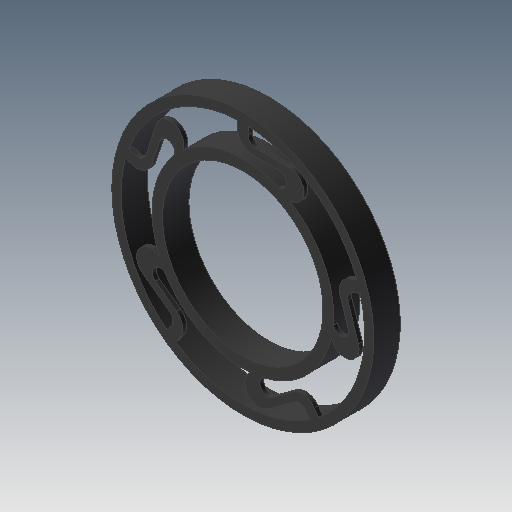
# Autodesk Inventor part: 01_Autofocus_CCTV12mm_spring_1
Saved by Autodesk Inventor 2019.4 (Build 234330000, 330)
## iProperties
Created: 2020-10-23
Part Number: 01_Autofocus_CCTV12mm_spring_1
Material: Generic
Document SubType Name: Modeling
Designer: diederichbenedict
Density: 1 g/cm^3
Appearance: Default
Author: diederichbenedict
Autodesk Inventor part; units mm, degrees
ref_plane "YZ Plane" through (0, 0, 0) normal (1, 0, 0) x (0, 1, 0)
ref_plane "XZ Plane" through (0, 0, 0) normal (0, 1, 0) x (-1, 0, 0)
ref_plane "XY Plane" through (0, 0, 0) normal (0, 0, 1) x (1, 0, 0)
ref_plane "Work Plane1" through (-22.2084, -34.255, 31.6599) normal (0, 0, 1) x (-1, 0, 0)
sketch "Sketch1" plane through (-22.2084, -34.255, 31.6599) normal (0, 0, 1) x (-1, 0, 0)
  circle A0 centre (0, 0) radius 10.2 construction
  circle A1 centre (0, 0) radius 9.25 projected
  circle A2 centre (0, 0) radius 6 projected
  circle A3 centre (0, 0) radius 6.1
  circle A4 centre (0, 0) radius 6.9
  circle A5 centre (0, 0) radius 9.95
  point P0 (-22.2084, -34.255)
  dimension "d0" = 12.2
  dimension "d1" = 0.8
  dimension "d10" = 19.9
  constraints: 3 centre point, 2 coincident
  measures "d0" diameter of A3
  measures "d1" radial gap between concentric circles of A3 A4
  measures "d10" diameter of A5
extrude "Extrusion1" add sketch "Sketch1" along normal blind 2 contours A4 | A5
sketch "Sketch2" plane through (-22.2084, -34.255, 33.6599) normal (0, 0, 1) x (1, 0, 0)
  circle A0 centre (0, 0) radius 6.1 construction
  circle A1 centre (0, 0) radius 6.9 construction
  circle A2 centre (0, 0) radius 9.25 construction
  circle A3 centre (0, 0) radius 9.25 construction
  line L0 (0.1042, 9.2494) -> (0.1042, 8.4994) construction
  circle A4 centre (0, 0) radius 6.9 construction
  line L1 (2.7219, 7.5216) -> (0.0969, 7.5216) construction
  line L2 (0.0969, 7.5216) -> (0.0969, 6.8993) construction
  line L3 (2.7219, 7.5216) -> (0.7649, 7.5216)
  line L4 (0.4969, 6.9) -> (0.4969, 6.8821)
  line L5 (3.5597, 8.0734) -> (0.9724, 8.0734)
  line L6 (0.4, 8.6458) -> (0.4, 9.2413)
  arc A5 (0.4969, 6.8821) -> (0.4969, 6.8821) centre (1.2774, -5.4017) ccw
  line L7 (-16.3817, 34.255) -> (28.6401, 34.255) projected
  arc A6 (3.5597, 5.9109) -> (3.5597, 8.0734) centre (3.5597, 6.9921) ccw
  arc A7 (2.7219, 6.3404) -> (2.7219, 7.5216) centre (2.7219, 6.931) ccw
  line L8 (-0.4, 9.0413) -> (-0.4, 9.2413)
  arc A8 (3.5597, 5.9109) -> (2.7219, 6.3404) centre (0, 0) ccw
  arc A9 (0.4, 9.2413) -> (-0.4, 9.2413) centre (0, 0) ccw
  arc A10 (3.5597, 5.9109) -> (2.3926, 6.4719) centre (0, 0) ccw construction
  arc A11 (0.4, 8.6458) -> (0.9724, 8.0734) centre (0.9724, 8.6458) ccw
  line L9 (22.2084, -18.791) -> (22.2084, 43.096) projected
  arc A12 (-0.4, 8.6864) -> (0.7649, 7.5216) centre (0.7649, 8.6864) ccw
  line L10 (-0.4, 9.0413) -> (-0.4, 8.6864)
  point P0 (22.2084, 34.255)
  point P1 (-2.5828, 8.8821)
  point P2 (-2.5828, 8.8821)
  point P3 (3.5023, 7.5216)
  dimension "d30" = 0.4
  dimension "d31" = 0.4
  constraints: 20 point on circle, 18 end point, 8 centre point, 6 tangent, 4 coincident, 2 horizontal, 2 parallel, 2 vertical, 1 concentric, 1 perpendicular, 1 point on line, 23 other
  measures "d30" distance from line of L8 A0.centre
  measures "d31" distance from line of A0.centre L6
extrude "Extrusion2" add sketch "Sketch2" against normal blind 0.3 contours L3 A12 L10 L8 A9 L6 A11 L5 A6 A5 A7 | A5 A6 A8 A7 picked at (3.3996, 6.4482)
pattern_circular "Circular Pattern1" count 5 over 360 about axis through (-22.2084, -34.255, 31.6599) along (0, 0, 1) of "Extrusion2"
equation "\"d30\" = d_1"
equation "\"d31\" = d_1"
equation "\"d_1\" = 0.4"
body "Solid1"
